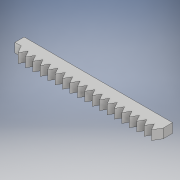
# Autodesk Inventor part: Backdrop Lateral Gear
Saved by Autodesk Inventor 2018 (Build 220112000, 112)
## iProperties
Created: 2018-12-13
Part Number: Backdrop Lateral Gear
Material: Generic
Document SubType Name: Modeling
Designer: F8PLTW
Density: 1 g/cm^3
Appearance: Default
Author: F8PLTW
Autodesk Inventor part; units mm, degrees
ref_plane "YZ Plane" through (0, 0, 0) normal (1, 0, 0) x (0, 1, 0)
ref_plane "XZ Plane" through (0, 0, 0) normal (0, 1, 0) x (-1, 0, 0)
ref_plane "XY Plane" through (0, 0, 0) normal (0, 0, 1) x (1, 0, 0)
sketch "Sketch1" plane through (0, 0, 0) normal (0, 0, 1) x (1, 0, 0)
  line L0 (-14.4276, 6.3576) -> (36.3724, 6.3576)
  line L1 (36.3724, 6.3576) -> (36.3724, 3.1826)
  line L2 (36.3724, 3.1826) -> (-14.4276, 3.1826)
  line L3 (-14.4276, 3.1826) -> (-14.4276, 6.3576)
  point P0 (0, 0)
  dimension "d0" = 50.8
  dimension "d1" = 3.175
  constraints: 8 end point, 2 parallel, 1 horizontal, 1 perpendicular
  measures "d0" distance of L1.end L2.end
  measures "d1" distance of L0.end L1.end
extrude "Extrusion1" add sketch "Sketch1" along normal blind 3.175
sketch "Sketch2" plane through (-14.4276, 6.3576, 0) normal (0, 1, 0) x (1, 0, 0)
  line L0 (50.8, -3.175) -> (0, -3.175) projected
  line L1 (50.8, -3.175) -> (49.3268, -5.7267)
  line L2 (49.3268, -5.7267) -> (47.8536, -3.175)
  line L3 (47.8536, -3.175) -> (50.8, -3.175)
  line L4 (48.26, -3.175) -> (46.7868, -5.7267)
  line L5 (46.7868, -5.7267) -> (45.3136, -3.175)
  line L6 (45.3136, -3.175) -> (48.26, -3.175)
  line L7 (45.72, -3.175) -> (44.2468, -5.7267)
  line L8 (44.2468, -5.7267) -> (42.7736, -3.175)
  line L9 (42.7736, -3.175) -> (45.72, -3.175)
  line L10 (43.18, -3.175) -> (41.7068, -5.7267)
  line L11 (41.7068, -5.7267) -> (40.2336, -3.175)
  line L12 (40.2336, -3.175) -> (43.18, -3.175)
  line L13 (40.64, -3.175) -> (39.1668, -5.7267)
  line L14 (39.1668, -5.7267) -> (37.6936, -3.175)
  line L15 (37.6936, -3.175) -> (40.64, -3.175)
  line L16 (38.1, -3.175) -> (36.6268, -5.7267)
  line L17 (36.6268, -5.7267) -> (35.1536, -3.175)
  line L18 (35.1536, -3.175) -> (38.1, -3.175)
  line L19 (35.56, -3.175) -> (34.0868, -5.7267)
  line L20 (34.0868, -5.7267) -> (32.6136, -3.175)
  line L21 (32.6136, -3.175) -> (35.56, -3.175)
  line L22 (33.02, -3.175) -> (31.5468, -5.7267)
  line L23 (31.5468, -5.7267) -> (30.0736, -3.175)
  line L24 (30.0736, -3.175) -> (33.02, -3.175)
  line L25 (30.48, -3.175) -> (29.0068, -5.7267)
  line L26 (29.0068, -5.7267) -> (27.5336, -3.175)
  line L27 (27.5336, -3.175) -> (30.48, -3.175)
  line L28 (27.94, -3.175) -> (26.4668, -5.7267)
  line L29 (26.4668, -5.7267) -> (24.9936, -3.175)
  line L30 (24.9936, -3.175) -> (27.94, -3.175)
  line L31 (25.4, -3.175) -> (23.9268, -5.7267)
  line L32 (23.9268, -5.7267) -> (22.4536, -3.175)
  line L33 (22.4536, -3.175) -> (25.4, -3.175)
  line L34 (22.86, -3.175) -> (21.3868, -5.7267)
  line L35 (21.3868, -5.7267) -> (19.9136, -3.175)
  line L36 (19.9136, -3.175) -> (22.86, -3.175)
  line L37 (20.32, -3.175) -> (18.8468, -5.7267)
  line L38 (18.8468, -5.7267) -> (17.3736, -3.175)
  line L39 (17.3736, -3.175) -> (20.32, -3.175)
  line L40 (17.78, -3.175) -> (16.3068, -5.7267)
  line L41 (16.3068, -5.7267) -> (14.8336, -3.175)
  line L42 (14.8336, -3.175) -> (17.78, -3.175)
  line L43 (15.24, -3.175) -> (13.7668, -5.7267)
  line L44 (13.7668, -5.7267) -> (12.2936, -3.175)
  line L45 (12.2936, -3.175) -> (15.24, -3.175)
  line L46 (12.7, -3.175) -> (11.2268, -5.7267)
  line L47 (11.2268, -5.7267) -> (9.7536, -3.175)
  line L48 (9.7536, -3.175) -> (12.7, -3.175)
  line L49 (10.16, -3.175) -> (8.6868, -5.7267)
  line L50 (8.6868, -5.7267) -> (7.2136, -3.175)
  line L51 (7.2136, -3.175) -> (10.16, -3.175)
  line L52 (7.62, -3.175) -> (6.1468, -5.7267)
  line L53 (6.1468, -5.7267) -> (4.6736, -3.175)
  line L54 (4.6736, -3.175) -> (7.62, -3.175)
  line L55 (5.08, -3.175) -> (3.6068, -5.7267)
  line L56 (3.6068, -5.7267) -> (2.1336, -3.175)
  line L57 (2.1336, -3.175) -> (5.08, -3.175)
  point P0 (14.4276, 0)
  point P1 (49.3268, -4.0256)
  dimension "d4" = 2.9464
  dimension "d7" = 2.54
  constraints: 114 end point, 1 horizontal, 1 point on line, 115 other
  measures "d4" distance of L0.start L2.end
  measures "d7" distance of L0.start L4.start
extrude "Extrusion2" add sketch "Sketch2" against normal blind 3.175
body "Solid1"
